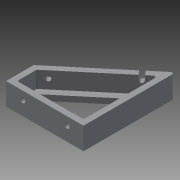
# Autodesk Inventor part: oled_halterung_W162_rechts
Saved by Autodesk Inventor 2015 (Build 190159000, 159)
## iProperties
Created: 2014-11-18
Part Number: oled_halterung_W162_rechts
Material: Generisch
Document SubType Name: Modeling
Designer: Zephram
Density: 1 g/cm^3
Appearance: Vorgabe
Author: Zephram
Autodesk Inventor part; units mm, degrees
ref_plane "YZ Plane" through (0, 0, 0) normal (1, 0, 0) x (0, 1, 0)
ref_plane "XZ Plane" through (0, 0, 0) normal (0, 1, 0) x (-1, 0, 0)
ref_plane "XY Plane" through (0, 0, 0) normal (0, 0, 1) x (1, 0, 0)
sketch "Skizze1" plane through (0, 0, 0) normal (0, 0, 1) x (1, 0, 0)
  line L0 (0, 0) -> (0, 50.2422)
  line L1 (0, 50.2422) -> (-42, 15)
  line L2 (-42, 15) -> (-42, 0)
  line L3 (-42, 0) -> (0, 0)
  line L4 (-6.5, 6.5) -> (-6.5, 36.3029)
  line L5 (-6.5, 36.3029) -> (-35.5, 11.969)
  line L6 (-35.5, 11.969) -> (-35.5, 6.5)
  line L7 (-35.5, 6.5) -> (-6.5, 6.5)
  dimension "d0" = 130
  dimension "d1" = 15
  dimension "d2" = 42
  dimension "d3" = 6.5
  dimension "d4" = 6.5
  dimension "d6" = 6.5
  dimension "d7" = 6.5
  constraints: 16 end point, 4 parallel, 2 vertical, 1 perpendicular
  measures "d0" angle of L2 L1
  measures "d1" distance of L2.end L1.end
  measures "d2" distance between parallel lines of L0 L2
  measures "d3" distance between parallel lines of L3 L7
  measures "d4" distance between parallel lines of L0 L4
  measures "d6" distance between parallel lines of L2 L6
  measures "d7" distance between parallel lines of L5 L1
extrude "Extrusion1" add sketch "Skizze1" along normal blind 12
sketch "Skizze2" plane through (0, 0, 12) normal (0, 0, 1) x (1, 0, 0)
  line L0 (-3, 43.8087) -> (-3, 3)
  line L1 (-3, 3) -> (-39, 3)
  line L2 (-39, 3) -> (-39, 13.6011)
  line L3 (-39, 13.6011) -> (-3, 43.8087)
  line L4 (-42, 0) -> (0, 0) projected
  line L5 (-42, 15) -> (-42, 0) projected
  line L6 (0, 50.2422) -> (-42, 15) projected
  line L7 (0, 0) -> (0, 50.2422) projected
  dimension "d10" = 3
  dimension "d11" = 3
  dimension "d12" = 3
  dimension "d13" = 3
  constraints: 8 end point, 4 parallel, 1 vertical
  measures "d10" distance between parallel lines of L5 L2
  measures "d11" distance between parallel lines of L7 L0
  measures "d12" distance between parallel lines of L4 L1
  measures "d13" distance between parallel lines of L6 L3
extrude "Extrusion2" cut sketch "Skizze2" against normal blind 9 contours L0 L1 L2 L3
sketch "Skizze3" plane through (-39, 3, 12) normal (0, 1, 0) x (1, 0, 0)
  line L0 (39, 12) -> (39, 0) projected
  line L1 (39, 0) -> (36, 0) projected
  line L2 (36, 0) -> (36, 9) projected
  line L3 (36, 9) -> (0, 9) projected
  line L4 (0, 9) -> (0, 0) projected
  line L5 (0, 0) -> (-3, 0) projected
  line L6 (-3, 0) -> (-3, 12) projected
  line L7 (-3, 12) -> (39, 12) projected
  line L8 (36, 0) -> (0, 0) projected
  line L9 (0, 4.5) -> (36, 4.5)
  point P0 (6, 4.5)
  point P1 (30, 4.5)
  dimension "d17" = 6
  dimension "d18" = 6
  constraints: 2 end point, 2 midpoint, 2 point on line
  measures "d17" distance from line of L4 point (6, 4.5)
  measures "d18" distance from line of L2 point (30, 4.5)
hole "Bohrung1" at (-33, 3, 7.5) at (-9, 3, 7.5) direction (0, -1, 0) diameter 2.7 depth 8 tip angle 118
fillet "Rundung2" radius 1 9 edges at (-6.5, 6.5, 1.5) (-3, 3, 7.5) (0, 50.2422, 6) (-6.5, 36.3029, 1.5) (-3, 43.8087, 7.5) (-39, 13.6011, 7.5) (-35.5, 11.969, 1.5) (-35.5, 6.5, 1.5) (-39, 3, 7.5)
sketch "Skizze4" plane through (-38.6428, 13.9008, 3) normal (0.6427876, -0.7660444, 0) x (0.7660444, 0.6427876, 0)
  line L0 (50.4446, -3) -> (-4.3825, -3) projected
  line L1 (-4.3825, -3) -> (-4.3825, 9) projected
  line L2 (-4.3825, 9) -> (0, 9) projected
  line L3 (0, 0) -> (0, 9) projected
  line L4 (0, 0) -> (44.3838, 0) projected
  line L5 (44.3838, 0) -> (44.3838, 9) projected
  line L6 (0, 9) -> (44.3838, 9) projected
  line L7 (50.4446, 9) -> (50.4446, -3) projected
  line L8 (44.3838, 9) -> (50.4446, 9) projected
  point P0 (20.6668, -3)
  point P1 (4, 5)
  point P2 (40, 6.5)
  dimension "d27" = 4
  dimension "d28" = 4
  dimension "d29" = 2.5
  dimension "d30" = 40
  dimension "d31" = 4.3838
  measures "d27" distance from line of L3 point (4, 5)
  measures "d28" distance from line of L6 point (4, 5)
  measures "d29" distance from line of L6 point (40, 6.5)
  measures "d30" distance from line of point (40, 6.5) L3
  measures "d31" distance from line of L5 point (40, 6.5)
hole "Bohrung2" at (-35.5786, 16.472, 8) at (-8.001, 39.6123, 9.5) direction (-0.6427876, 0.7660444, 0) diameter 2.5 depth 8 tip angle 118
sketch "Skizze5" plane through (-38.6428, 13.9008, 3) normal (0.6427876, -0.7660444, 0) x (0.7660444, 0.6427876, 0)
  circle A0 centre (40, 6.5) radius 1.25 projected
  line L0 (41.25, 6.5) -> (41.25, 9)
  line L1 (50.8174, 9) -> (-1.8652, 9) projected
  line L2 (38.75, 9) -> (38.75, 6.5)
  point P0 (20.6668, -3)
  constraints: 4 end point, 2 point on circle, 2 point on line, 2 tangent, 1 vertical
extrude "Extrusion3" cut sketch "Skizze5" against normal blind 16.75 contours A0 L2 L1 L0
